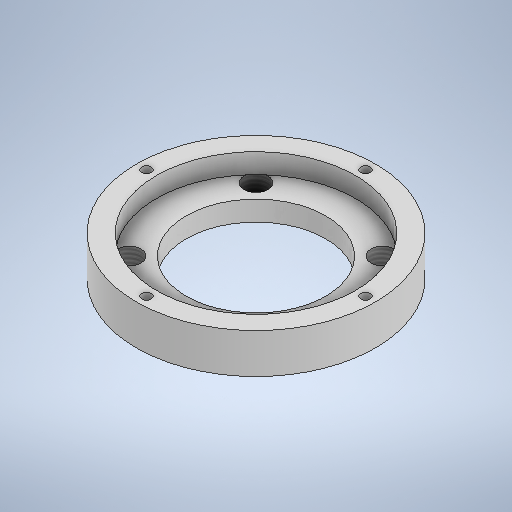
# Autodesk Inventor part: Placeholderjointouterring
Saved by Autodesk Inventor 2025.2 (Build 292293000, 293)
## iProperties
Created: 2026-03-22
Part Number: Placeholderjointouterring
Material: Generic
Document SubType Name: Modeling
Designer: hp
Density: 1 g/cm^3
Appearance: Default
Author: hp
Autodesk Inventor part; units mm, degrees
ref_plane "YZ Plane" through (0, 0, 0) normal (1, 0, 0) x (0, 1, 0)
ref_plane "XZ Plane" through (0, 0, 0) normal (0, 1, 0) x (-1, 0, 0)
ref_plane "XY Plane" through (0, 0, 0) normal (0, 0, 1) x (1, 0, 0)
sketch "Sketch1" plane through (0, 0, 0) normal (0, 1, 0) x (-1, 0, 0)
  circle A0 centre (0, 0) radius 25
  circle A1 centre (0, 0) radius 30
  circle A2 centre (0, 0) radius 17.5
  line L0 (0, 0) -> (25, 0) construction
  circle A3 centre (17.6777, -17.6777) radius 2
  circle A4 centre (17.6777, 17.6777) radius 2
  circle A5 centre (-17.6777, 17.6777) radius 2
  circle A6 centre (-17.6777, -17.6777) radius 2
  point P0 (0, -27.5)
  point P1 (0, -27.5)
  point P2 (27.5, 0)
  point P3 (-27.5, 0)
  point P4 (0, 27.5)
  dimension "d0" = 50
  dimension "d1" = 60
  dimension "d17" = 27.5
  dimension "d18" = 27.5
  dimension "d19" = 27.5
  dimension "d20" = 27.5
  dimension "d28" = 35
  dimension "d30" = 4
  dimension "d33" = 360
  constraints: 7 centre point, 4 coincident, 2 end point, 1 horizontal, 9 other
  measures "d0" diameter of A0
  measures "d1" diameter of A1
  measures "d17" distance of point (0, 0) point (27.5, 0)
  measures "d18" distance of point (-27.5, 0) point (0, 0)
  measures "d19" distance of point (0, 0) point (0, 27.5)
  measures "d20" distance of point (0, -27.5) point (0, 0)
  measures "d28" diameter of A2
  measures "d30" diameter of A3
extrude "Extrusion1" add sketch "Sketch1" along normal blind 5 contours A0 A4 | A3 A0 | A0 A5 | A6 A0 | A1 picked at (18.1752, 18.1125) picked at (18.1752, -18.1125) picked at (-18.083, 18.1995) picked at (-18.083, -18.1995)
extrude "Extrusion2" add sketch "Sketch1" against normal blind 5 contours A0 A3 A6 A5 A4 | A4 A0 | A0 A4 | A3 A0 | A0 A3 | A5 A0 | A0 A5 | A6 A0 | A0 A6 | A1
hole "Hole2" at (0, 0, -27.5) at (-27.5, 0, 0) at (27.5, 0, 0) at (0, 0, 27.5) direction (0, 1, 0) diameter 2.45 end through all
sketch "Sketch2" plane through (0, -5, 0) normal (0, -1, 0) x (1, 0, 0)
  circle A0 centre (0, 0) radius 22.5
  line L0 (0, 0) -> (15.9099, 15.9099)
  line L1 (0, 0) -> (22.5, 0) construction
  circle A1 centre (15.9099, 15.9099) radius 3
  circle A2 centre (-15.9099, 15.9099) radius 3
  circle A3 centre (-15.9099, -15.9099) radius 3
  circle A4 centre (15.9099, -15.9099) radius 3
  dimension "d35" = 45
  dimension "d36" = 45
  dimension "d37" = 6
  dimension "d40" = 360
  constraints: 4 centre point, 4 end point, 2 coincident, 1 equal length, 1 horizontal, 12 other
  measures "d36" angle of L1 L0
  measures "d37" diameter of A1
extrude "Extrusion3" cut sketch "Sketch2" against normal blind 5 contours A1 L0 A0 | A0 A1 | A4 A0 | A0 A4 | L0 A1 A0 | A3 A0 | A0 A3 | A2 A0 | A0 A2
thread "Thread1" size "M6x1" class "6H" standard "ISO Metric profile" full length
thread "Thread2" size "M6x1" class "6H" standard "ISO Metric profile" full length
thread "Thread3" size "M6x1" class "6H" standard "ISO Metric profile" full length
thread "Thread4" size "M6x1" class "6H" standard "ISO Metric profile" full length
body "Solid1"
